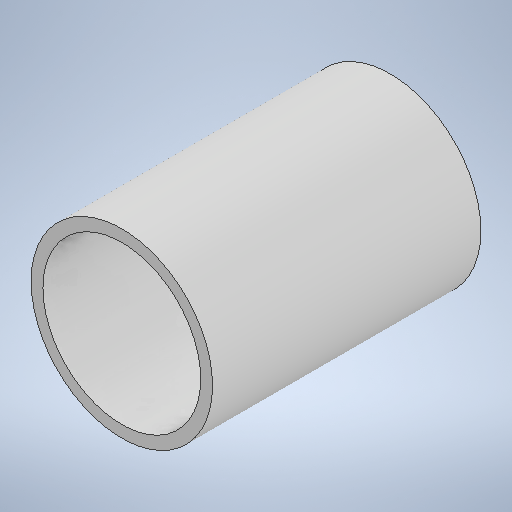
# Autodesk Inventor part: tuleja_dys
Saved by Autodesk Inventor 2025 (Build 290162000, 162)
## iProperties
Created: 2025-05-31
Part Number: tuleja_dys
Material: Ogólny
Document SubType Name: Modeling
Designer: tjaku
Density: 1 g/cm^3
Appearance: Domyślna
Author: tjaku
Autodesk Inventor part; units mm, degrees
ref_plane "YZ Plane" through (0, 0, 0) normal (1, 0, 0) x (0, 1, 0)
ref_plane "XZ Plane" through (0, 0, 0) normal (0, 1, 0) x (-1, 0, 0)
ref_plane "XY Plane" through (0, 0, 0) normal (0, 0, 1) x (1, 0, 0)
sketch "Szkic2" plane through (0, 0, 0) normal (0, 0, 1) x (1, 0, 0)
  circle A0 centre (0, 0) radius 10
  circle A1 centre (0, 0) radius 11.5
  dimension "d5" = 20
  dimension "d6" = 23
  constraints: 2 centre point, 2 coincident
  measures "d5" diameter of A0
  measures "d6" diameter of A1
extrude "Wyciągnięcie proste2" add sketch "Szkic2" along normal blind 34.025
